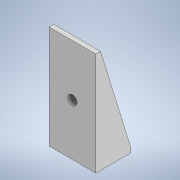
# Autodesk Inventor part: MM3_vertical
Saved by Autodesk Inventor 2021 (Build 250183000, 183)
## iProperties
Created: 2021-02-23
Part Number: MM3_vertical
Material: Generic
Document SubType Name: Modeling
Designer: dsdan
Density: 1 g/cm^3
Appearance: Default
Author: dsdan
Autodesk Inventor part; units mm, degrees
ref_plane "YZ Plane" through (0, 0, 0) normal (1, 0, 0) x (0, 1, 0)
ref_plane "XZ Plane" through (0, 0, 0) normal (0, 1, 0) x (-1, 0, 0)
ref_plane "XY Plane" through (0, 0, 0) normal (0, 0, 1) x (1, 0, 0)
sketch "Sketch2" plane through (0, 0, 0) normal (1, 0, 0) x (0, 1, 0)
  line L0 (0, 0) -> (44.2, 0)
  line L1 (44.2, 0) -> (44.2, -2)
  line L2 (44.2, -2) -> (2, -15)
  line L3 (2, -15) -> (0, -15)
  line L4 (0, -15) -> (0, 0)
  dimension "d0" = 44.2
  dimension "d1" = 2
  dimension "d2" = 2
  dimension "d3" = 15
  constraints: 10 end point, 2 perpendicular, 1 horizontal, 1 parallel
  measures "d0" distance of L0.start L0.end
  measures "d1" distance of L0.end L1.end
  measures "d2" distance of L2.end L3.end
  measures "d3" distance of L3.end L0.start
extrude "Extrusion1" add sketch "Sketch2" along normal blind 20
sketch "Sketch3" plane through (0, 0, -15) normal (0, -1, 0) x (1, 0, 0)
  line L0 (0, 15) -> (20, 15) projected
  line L1 (0, 15) -> (20, 0) construction
  line L2 (0, 0) -> (0, 13) projected
  line L3 (20, 15) -> (0, 0) construction
  circle A0 centre (10, 7.5) radius 2
  dimension "d6" = 4
  constraints: 4 end point, 1 centre point, 1 midpoint
  measures "d6" diameter of A0
extrude "Extrusion2" cut sketch "Sketch3" against normal through all
sketch "Sketch4" plane through (0, 0, 0) normal (0, 0, 1) x (1, 0, 0)
  line L0 (20, 2) -> (20, 44.2) projected
  line L1 (20, 44.2) -> (0, 0) construction
  line L2 (20, 0) -> (20, 2) projected
  line L3 (0, 2) -> (0, 44.2) projected
  line L4 (20, 0) -> (0, 44.2) construction
  circle A0 centre (10, 22.1) radius 2
  dimension "d9" = 4
  constraints: 4 end point, 1 centre point, 1 coincident, 1 midpoint
  measures "d9" diameter of A0
extrude "Extrusion3" cut sketch "Sketch4" against normal through all
body "Solid1"
